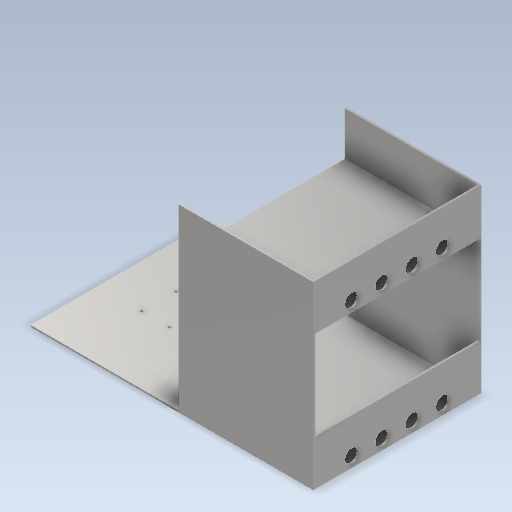
# Autodesk Inventor part: Valves_Pump Holder
Saved by Autodesk Inventor 2020 (Build 240168000, 168)
## iProperties
Created: 2020-08-10
Part Number: Valves_Pump Holder
Material: Generic
Document SubType Name: Modeling
Designer: Abbas
Density: 1 g/cm^3
Appearance: Default
Author: Abbas
Autodesk Inventor part; units mm, degrees
ref_plane "YZ Plane" through (0, 0, 0) normal (1, 0, 0) x (0, 1, 0)
ref_plane "XZ Plane" through (0, 0, 0) normal (0, 1, 0) x (-1, 0, 0)
ref_plane "XY Plane" through (0, 0, 0) normal (0, 0, 1) x (1, 0, 0)
sketch "Sketch1" plane through (0, 0, 0) normal (1, 0, 0) x (0, 1, 0)
  line L0 (10.5163, 293.3597) -> (7.5163, 293.3597)
  line L1 (7.5163, 293.3597) -> (7.5163, 43.3597)
  line L2 (7.5163, 43.3597) -> (10.5163, 43.3597)
  line L3 (10.5163, 43.3597) -> (10.5163, 293.3597)
  line L4 (10.5163, 293.3597) -> (7.5163, 43.3597) construction
  line L5 (7.5163, 293.3597) -> (10.5163, 43.3597) construction
  line L6 (7.5163, 46.3597) -> (-192.4837, 46.3597)
  line L7 (-192.4837, 46.3597) -> (-192.4837, 43.3597)
  line L8 (-192.4837, 43.3597) -> (7.5163, 43.3597)
  line L9 (7.5163, 43.3597) -> (7.5163, 46.3597)
  line L10 (7.5163, 46.3597) -> (-192.4837, 43.3597) construction
  line L11 (-192.4837, 46.3597) -> (7.5163, 43.3597) construction
  line L12 (7.5163, 168.3597) -> (-42.4837, 168.3597)
  line L13 (7.5163, 168.3597) -> (57.5163, 168.3597) construction
  line L14 (7.5163, 290.3597) -> (-192.4837, 290.3597)
  line L15 (-192.4837, 290.3597) -> (-192.4837, 293.3597)
  line L16 (-192.4837, 293.3597) -> (7.5163, 293.3597)
  line L17 (7.5163, 290.3597) -> (-192.4837, 293.3597) construction
  line L18 (-192.4837, 290.3597) -> (7.5163, 293.3597) construction
  line L19 (-189.4837, 290.3597) -> (-192.4837, 290.3597)
  line L20 (-192.4837, 290.3597) -> (-192.4837, 46.3597)
  line L21 (-192.4837, 46.3597) -> (-189.4837, 46.3597)
  line L22 (-189.4837, 46.3597) -> (-189.4837, 290.3597)
  line L23 (-189.4837, 290.3597) -> (-192.4837, 46.3597) construction
  line L24 (-192.4837, 290.3597) -> (-189.4837, 46.3597) construction
  point P0 (0, 0)
  point P1 (9.0163, 168.3597)
  point P2 (-92.4837, 44.8597)
  point P3 (-92.4837, 291.8597)
  point P4 (-189.2359, -83.872)
  point P5 (7.5163, 290.3597)
  point P6 (7.5163, 46.3597)
  point P7 (-190.9837, 168.3597)
  point P8 (-189.4837, 46.3597)
  point P9 (-189.4837, 290.3597)
  dimension "d0" = 3
  dimension "d1" = 250
  dimension "d2" = 200
  dimension "d3" = 3
  dimension "d4" = 50
  dimension "d5" = 180
  dimension "d19" = 244
  constraints: 50 end point, 9 midpoint, 6 parallel, 5 horizontal, 4 symmetric about line, 3 perpendicular, 1 collinear
  measures "d0" distance of L2.end L1.end
  measures "d1" distance of L1.end L0.end
  measures "d2" distance of L1.end L7.end
  measures "d3" distance of L7.end L6.end
  measures "d4" distance of L12.start L12.end
  measures "d5" angle of L12 L13
  measures "d19" distance of L14.end L20.end
extrude "Extrusion1" add sketch "Sketch1" against normal blind 200 contours L3 L2 L1 L0 | L1 L14 L15 L16 | L8 L7 L6 L1 | L22 L6 L20 L14
sketch "Sketch3" plane through (-200, 0, 0) normal (-1, 0, 0) x (0, 0, 1)
  line L0 (43.3597, -189.4837) -> (293.3597, -189.4837)
  line L1 (293.3597, -189.4837) -> (293.3597, -192.4837)
  line L2 (293.3597, -192.4837) -> (43.3597, -192.4837)
  line L3 (43.3597, -192.4837) -> (43.3597, -189.4837)
  line L4 (43.3597, -189.4837) -> (293.3597, -192.4837) construction
  line L5 (293.3597, -189.4837) -> (43.3597, -192.4837) construction
  line L6 (46.3597, -189.4837) -> (290.3597, -189.4837) projected
  line L7 (290.3597, -189.4837) -> (46.3597, -189.4837)
  line L8 (290.3597, -189.4837) -> (534.3597, -189.4837) construction
  point P0 (0, 0)
  point P1 (168.3597, -190.9837)
  point P2 (168.3597, -189.4837)
  dimension "d20" = 250
  dimension "d21" = 3
  dimension "d22" = 244
  dimension "d23" = 180
  constraints: 16 end point, 4 midpoint, 3 equal length, 2 horizontal, 1 collinear, 1 perpendicular
  measures "d20" distance of L1.end L2.end
  measures "d21" distance of L0.end L1.end
  measures "d22" distance of L6.end L6.start
  measures "d23" angle of L7 L8
extrude "Extrusion3" add sketch "Sketch3" along normal blind 220
sketch "Sketch7" plane through (0, -189.4837, 290.3597) normal (0, 1, 0) x (1, 0, 0)
  line L0 (-200, 247) -> (-420, 247) projected
  line L1 (-200, -3) -> (-420, -3) projected
  line L2 (-420, -3) -> (-420, 247) projected
  point P0 (0, 290.3597)
  point P1 (-355, 97)
  point P2 (-355, 147.8)
  point P3 (-313.725, 147.8)
  point P4 (-313.725, 97)
  point P5 (-200, 244)
  point P6 (-200, 0)
  point P7 (-350, 369)
  point P8 (-350, -125)
  dimension "d53" = 50.8
  dimension "d54" = 50.8
  dimension "d55" = 41.275
  dimension "d56" = 41.275
  dimension "d59" = 100
  dimension "d60" = 100
  dimension "d61" = 65
  dimension "d62" = 65
  constraints: 2 other
  measures "d53" distance of point (-355, 147.8) point (-355, 97)
  measures "d54" distance of point (-313.725, 147.8) point (-313.725, 97)
  measures "d55" distance of point (-355, 147.8) point (-313.725, 147.8)
  measures "d56" distance of point (-355, 97) point (-313.725, 97)
  measures "d61" distance from line of L2 point (-355, 147.8)
  measures "d62" distance from line of L2 point (-355, 97)
hole "Hole1" at (-355, -189.4837, 193.3597) at (-355, -189.4837, 142.5597) at (-313.725, -189.4837, 142.5597) at (-313.725, -189.4837, 193.3597) direction (0, -1, 0) diameter 4.572 depth 26 tip angle 118
sketch "Sketch8" plane through (0, 10.5163, 293.3597) normal (0, 1, 0) x (1, 0, 0)
  line L0 (-3, 250) -> (0, 250)
  line L1 (0, 250) -> (0, 0)
  line L2 (0, 0) -> (-3, 0)
  line L3 (-3, 0) -> (-3, 250)
  line L4 (-3, 250) -> (0, 0) construction
  line L5 (0, 250) -> (-3, 0) construction
  line L6 (0, 250) -> (0, 0) projected
  line L7 (-200, 250) -> (-3, 250)
  line L8 (-3, 250) -> (-3, 247)
  line L9 (-3, 247) -> (-200, 247)
  line L10 (-200, 247) -> (-200, 250)
  line L11 (-200, 250) -> (-3, 247) construction
  line L12 (-3, 250) -> (-200, 247) construction
  line L13 (-200, 3) -> (-3, 3)
  line L14 (-3, 3) -> (-3, 0)
  line L15 (-3, 0) -> (-200, 0)
  line L16 (-200, 0) -> (-200, 3)
  line L17 (-200, 3) -> (-3, 0) construction
  line L18 (-3, 3) -> (-200, 0) construction
  point P0 (0, 293.3597)
  point P1 (-1.5, 125)
  point P2 (0, 125)
  point P3 (-101.5, 248.5)
  point P4 (-101.5, 1.5)
  point P5 (-3, 3)
  dimension "d63" = 3
  dimension "d64" = 250
  dimension "d82" = 197
  dimension "d83" = 3
  dimension "d84" = 197
  dimension "d85" = 3
  constraints: 36 end point, 8 midpoint, 6 parallel, 3 horizontal, 3 perpendicular
  measures "d63" distance of L1.end L2.end
  measures "d64" distance of L0.end L1.end
  measures "d82" distance of L8.end L9.end
  measures "d83" distance of L0.start L8.end
  measures "d84" distance of L2.end L15.end
  measures "d85" distance of L2.end L13.end
extrude "Extrusion7" add sketch "Sketch8" along normal blind 65 contours L0 L1 L2 L3
sketch "Sketch9" plane through (0, 0, 0) normal (1, 0, 0) x (0, 0, -1)
  line L0 (-293.3597, 10.5163) -> (-43.3597, 10.5163) projected
  line L1 (-293.3597, 75.5163) -> (-293.3597, -192.4837) projected
  point P0 (0, 0)
  point P1 (-235.8597, 23.0163)
  point P2 (-190.8597, 23.0163)
  point P3 (-145.8597, 23.0163)
  point P4 (-100.8597, 23.0163)
  dimension "d74" = 12.5
  dimension "d75" = 12.5
  dimension "d76" = 12.5
  dimension "d77" = 12.5
  dimension "d78" = 45
  dimension "d79" = 45
  dimension "d80" = 45
  dimension "d81" = 57.5
  measures "d74" distance from line of L0 point (-235.86, 23.016)
  measures "d75" distance from line of L0 point (-190.86, 23.016)
  measures "d76" distance from line of L0 point (-145.86, 23.016)
  measures "d77" distance from line of L0 point (-100.86, 23.016)
  measures "d78" distance of point (-190.86, 23.016) point (-235.86, 23.016)
  measures "d79" distance of point (-145.86, 23.016) point (-190.86, 23.016)
  measures "d80" distance of point (-100.86, 23.016) point (-145.86, 23.016)
  measures "d81" distance from line of L1 point (-235.86, 23.016)
hole "Hole2" at (0, 23.0163, 235.8597) at (0, 23.0163, 190.8597) at (0, 23.0163, 145.8597) at (0, 23.0163, 100.8597) direction (-1, 0, 0) diameter 20 depth 26 tip angle 118
extrude "Extrusion8" add sketch "Sketch8" along normal blind 65 contours L3 L9 L10 L7 | L3 L15 L16 L13
sketch "Sketch10" plane through (0, -189.4837, 290.3597) normal (0, 1, 0) x (1, 0, 0)
  line L0 (-3, 0) -> (0, 0)
  line L1 (0, 0) -> (0, 244)
  line L2 (0, 244) -> (-3, 244)
  line L3 (-3, 244) -> (-3, 0)
  line L4 (-3, 0) -> (0, 244) construction
  line L5 (0, 0) -> (-3, 244) construction
  line L6 (0, 244) -> (0, 0) projected
  point P0 (0, 290.3597)
  point P1 (-1.5, 122)
  point P2 (0, 122)
  dimension "d89" = 3
  dimension "d90" = 244
  constraints: 12 end point, 4 midpoint, 2 parallel, 1 horizontal, 1 perpendicular
  measures "d89" distance of L2.end L1.end
  measures "d90" distance of L1.end L0.end
extrude "Extrusion9" add sketch "Sketch10" along normal blind 65
sketch "Sketch11" plane through (0, 0, 0) normal (1, 0, 0) x (0, 0, -1)
  line L0 (-290.3597, -189.4837) -> (-46.3597, -189.4837) projected
  line L1 (-293.3597, 75.5163) -> (-293.3597, -192.4837) projected
  point P0 (0, 0)
  point P1 (-235.8597, -176.9837)
  point P2 (-190.8597, -176.9837)
  point P3 (-145.8597, -176.9837)
  point P4 (-100.8597, -176.9837)
  dimension "d100" = 12.5
  dimension "d101" = 12.5
  dimension "d102" = 12.5
  dimension "d103" = 12.5
  dimension "d104" = 57.5
  dimension "d105" = 45
  dimension "d106" = 45
  dimension "d107" = 45
  measures "d100" distance from line of L0 point (-235.86, -176.984)
  measures "d101" distance from line of L0 point (-190.86, -176.984)
  measures "d102" distance from line of L0 point (-145.86, -176.984)
  measures "d103" distance from line of L0 point (-100.86, -176.984)
  measures "d104" distance from line of L1 point (-235.86, -176.984)
  measures "d105" distance of point (-190.86, -176.984) point (-235.86, -176.984)
  measures "d106" distance of point (-145.86, -176.984) point (-190.86, -176.984)
  measures "d107" distance of point (-100.86, -176.984) point (-145.86, -176.984)
hole "Hole3" at (0, -176.9837, 235.8597) at (0, -176.9837, 190.8597) at (0, -176.9837, 145.8597) at (0, -176.9837, 100.8597) direction (-1, 0, 0) diameter 20 depth 26 tip angle 118
body "Solid1"
